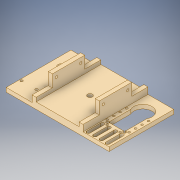
# Autodesk Inventor part: База
Saved by Autodesk Inventor 2019 (Build 230136000, 136)
## iProperties
Created: 2019-08-15
Part Number: База
Material: Пластик АБС
Document SubType Name: Modeling
Designer: Петров Иван
Density: 1.06 g/cm^3
Appearance: Гладкий — серовато-белый
Author: Петров Иван
Autodesk Inventor part; units mm, degrees
ref_plane "YZ Plane" through (0, 0, 0) normal (1, 0, 0) x (0, 1, 0)
ref_plane "XZ Plane" through (0, 0, 0) normal (0, 1, 0) x (-1, 0, 0)
ref_plane "XY Plane" through (0, 0, 0) normal (0, 0, 1) x (1, 0, 0)
sketch "Эскиз1" plane through (0, 0, 0) normal (0, 1, 0) x (-1, 0, 0)
  line L0 (-31.5, 40) -> (31.5, 40)
  line L1 (31.5, 40) -> (31.5, -40)
  line L2 (31.5, -40) -> (-31.5, -40)
  line L3 (-31.5, -40) -> (-31.5, 40)
  line L4 (-31.5, 40) -> (31.5, -40) construction
  line L5 (31.5, 40) -> (-31.5, -40) construction
  point P0 (0, 0)
  dimension "d0" = 63
  dimension "d1" = 80
  constraints: 12 end point, 2 midpoint, 2 parallel, 1 horizontal, 1 perpendicular
  measures "d0" distance of L1.end L2.end
  measures "d1" distance of L0.end L1.end
extrude "Выдавливание1" add sketch "Эскиз1" along normal blind 8
sketch "Эскиз2" plane through (0, 8, 0) normal (0, 1, 0) x (1, 0, 0)
  line L0 (-31.5, -40) -> (31.5, -40) projected
  line L1 (31.5, 40) -> (-31.5, 40) projected
  line L2 (-31.5, -40) -> (-26.5, -40)
  line L3 (-26.5, -40) -> (-26.5, 40)
  line L4 (-26.5, 40) -> (-31.5, 40)
  line L5 (-31.5, 40) -> (-31.5, -40)
  line L6 (31.5, -40) -> (31.5, 40) projected
  line L7 (31.5, 40) -> (26.5, 40)
  line L8 (26.5, 40) -> (26.5, -40)
  line L9 (26.5, -40) -> (31.5, -40)
  line L10 (31.5, -40) -> (31.5, 40)
  point P0 (0, 0)
  dimension "d4" = 5
  dimension "d5" = 5
  constraints: 16 end point, 4 parallel, 2 horizontal, 2 perpendicular, 2 point on line
  measures "d4" distance of L4.end L3.end
  measures "d5" distance of L9.end L8.end
extrude "Выдавливание2" add sketch "Эскиз2" along normal blind 20 contours L5 L1 L3 L0 | L8 L1 L6 L0
sketch "Эскиз3" plane through (-26.5, 8, 40) normal (1, 0, 0) x (0, 0, -1)
  line L0 (0, 0) -> (0, 20) projected
  line L1 (0, 0) -> (25, 0)
  line L2 (25, 0) -> (25, 14)
  line L3 (25, 14) -> (0, 14)
  line L4 (0, 14) -> (0, 0)
  circle A0 centre (25, 14) radius 1.5
  line L5 (80, 20) -> (0, 20) projected
  line L6 (40, 20) -> (40, 22.577)
  circle A1 centre (55, 14) radius 1.5
  point P0 (40, -8)
  dimension "d8" = 25
  dimension "d9" = 14
  dimension "d10" = 3
  constraints: 10 end point, 2 centre point, 2 parallel, 1 coincident, 1 horizontal, 1 midpoint, 1 perpendicular, 1 symmetric about line, 1 vertical, 1 other
  measures "d8" distance of L3.end L2.end
  measures "d9" distance of L2.end L1.end
  measures "d10" diameter of A0
extrude "Выдавливание3" cut sketch "Эскиз3" along normal blind 63.5 and the other way blind 5 contours A0 L2 L3 | L3 L2 A0 | A1
sketch "Эскиз4" plane through (0, 0, 0) normal (0, -1, 0) x (1, 0, 0)
  line L0 (31.5, -40) -> (31.5, 40) projected
  line L1 (31.5, -40) -> (63.5, -40)
  line L2 (63.5, -40) -> (63.5, 40)
  line L3 (63.5, 40) -> (31.5, 40)
  line L4 (31.5, 40) -> (31.5, -40)
  point P0 (0, 0)
  dimension "d15" = 32
  dimension "d16" = 80
  constraints: 8 end point, 2 parallel, 1 horizontal, 1 perpendicular
  measures "d15" distance of L3.end L2.end
  measures "d16" distance of L2.end L1.end
extrude "Выдавливание4" add sketch "Эскиз4" against normal blind 5
sketch "Эскиз5" plane through (0, 5, 0) normal (0, 1, 0) x (1, 0, 0)
  line L0 (34.2298, 0.6569) -> (31.9298, 0.6569)
  line L1 (34.2298, 0.6569) -> (34.2298, -0.7431)
  line L2 (31.9298, -0.7431) -> (34.2298, -0.7431)
  line L3 (31.9298, -7.3431) -> (31.9298, -0.7431)
  line L4 (34.2298, -7.3431) -> (31.9298, -7.3431)
  circle A0 centre (46.8802, 18.4564) radius 9.15
  circle A1 centre (46.8298, 18.4569) radius 1.5
  circle A2 centre (54.8298, -17.5431) radius 1.3
  circle A3 centre (60.3298, -4.0431) radius 1.3
  circle A4 centre (60.3298, -12.0431) radius 1.3
  circle A5 centre (60.3298, 3.9569) radius 1.3
  circle A6 centre (60.3298, 11.9569) radius 1.3
  circle A7 centre (38.8298, -17.5431) radius 1.3
  circle A8 centre (33.3298, -4.0431) radius 1.3
  circle A9 centre (33.3298, -12.0431) radius 1.3
  circle A10 centre (33.3298, 3.9569) radius 1.3
  circle A11 centre (33.3298, 11.9569) radius 1.3
  line L5 (46.7298, 29.4767) -> (46.7298, 28.9365)
  line L6 (39.8298, 29.4767) -> (46.7298, 29.4767)
  arc A12 (39.8298, 29.4767) -> (39.0798, 29.4255) centre (39.8298, 23.9569) ccw
  line L7 (39.0798, 26.9569) -> (39.0798, 29.4255)
  arc A13 (37.3298, 25.2069) -> (39.0798, 26.9569) centre (37.3298, 26.9569) ccw
  line L8 (36.8298, 25.2069) -> (37.3298, 25.2069)
  line L9 (36.8298, -12.3493) -> (36.8298, 25.2069)
  arc A14 (36.8298, -12.3493) -> (37.2219, -13.0376) centre (37.6298, -12.3493) ccw
  arc A15 (37.2219, -13.0376) -> (37.8353, -13.6509) centre (36.3298, -14.5431) ccw
  arc A16 (37.8353, -13.6509) -> (38.5235, -14.0431) centre (38.5235, -13.2431) ccw
  line L10 (55.136, -14.0431) -> (38.5235, -14.0431)
  arc A17 (55.136, -14.0431) -> (55.8243, -13.6509) centre (55.136, -13.2431) ccw
  arc A18 (56.4376, -13.0376) -> (55.8243, -13.6509) centre (57.3298, -14.5431) ccw
  arc A19 (55.8243, -13.6509) -> (56.4376, -13.0376) centre (57.3298, -14.5431) ccw
  line L11 (35.5069, 25.2069) -> (36.8298, 25.2069)
  arc A20 (35.5069, 25.2069) -> (35.3298, 23.9569) centre (39.8376, 23.9558) ccw
  line L12 (35.3298, 23.9569) -> (35.3298, 16.4569)
  line L13 (34.2298, 16.4569) -> (35.3298, 16.4569)
  line L14 (34.2298, 15.2569) -> (34.2298, 16.4569)
  line L15 (31.9298, 15.2569) -> (34.2298, 15.2569)
  line L16 (31.9298, 8.6569) -> (31.9298, 15.2569)
  line L17 (34.2298, 8.6569) -> (31.9298, 8.6569)
  line L18 (34.2298, 7.2569) -> (34.2298, 8.6569)
  line L19 (31.9298, 7.2569) -> (34.2298, 7.2569)
  line L20 (31.9298, 0.6569) -> (31.9298, 7.2569)
  line L21 (34.2298, 0.6569) -> (31.9298, 0.6569)
  line L22 (34.2298, -0.7431) -> (34.2298, 0.6569)
  line L23 (31.9298, -0.7431) -> (34.2298, -0.7431)
  line L24 (31.9298, -7.3431) -> (31.9298, -0.7431)
  line L25 (34.2298, -7.3431) -> (31.9298, -7.3431)
  line L26 (34.2298, -8.7431) -> (34.2298, -7.3431)
  line L27 (31.9298, -8.7431) -> (34.2298, -8.7431)
  line L28 (31.9298, -15.3431) -> (31.9298, -8.7431)
  line L29 (34.2298, -15.3431) -> (31.9298, -15.3431)
  line L30 (34.2298, -16.5629) -> (34.2298, -15.3431)
  arc A21 (34.2298, -16.5629) -> (34.31, -16.6431) centre (35.3298, -15.5431) ccw
  line L31 (35.5298, -16.6431) -> (34.31, -16.6431)
  line L32 (35.5298, -18.9431) -> (35.5298, -16.6431)
  line L33 (42.1298, -18.9431) -> (35.5298, -18.9431)
  line L34 (42.1298, -16.6431) -> (42.1298, -18.9431)
  line L35 (51.5298, -16.6431) -> (42.1298, -16.6431)
  line L36 (51.5298, -18.9431) -> (51.5298, -16.6431)
  line L37 (58.1298, -18.9431) -> (51.5298, -18.9431)
  line L38 (58.1298, -16.6431) -> (58.1298, -18.9431)
  line L39 (59.3496, -16.6431) -> (58.1298, -16.6431)
  arc A22 (59.3496, -16.6431) -> (59.4298, -16.5629) centre (58.3298, -15.5431) ccw
  line L40 (59.4298, -15.3431) -> (59.4298, -16.5629)
  line L41 (61.7298, -15.3431) -> (59.4298, -15.3431)
  line L42 (61.7298, -8.7431) -> (61.7298, -15.3431)
  line L43 (59.4298, -8.7431) -> (61.7298, -8.7431)
  line L44 (59.4298, -7.3431) -> (59.4298, -8.7431)
  line L45 (61.7298, -7.3431) -> (59.4298, -7.3431)
  line L46 (61.7298, -0.7431) -> (61.7298, -7.3431)
  line L47 (59.4298, -0.7431) -> (61.7298, -0.7431)
  line L48 (59.4298, 0.6569) -> (59.4298, -0.7431)
  line L49 (61.7298, 0.6569) -> (59.4298, 0.6569)
  line L50 (61.7298, 7.2569) -> (61.7298, 0.6569)
  line L51 (59.4298, 7.2569) -> (61.7298, 7.2569)
  line L52 (59.4298, 8.6569) -> (59.4298, 7.2569)
  line L53 (61.7298, 8.6569) -> (59.4298, 8.6569)
  line L54 (61.7298, 15.2568) -> (61.7298, 8.6569)
  line L55 (59.4305, 15.2569) -> (61.7298, 15.2568)
  line L56 (59.4306, 16.4569) -> (59.4305, 15.2569)
  line L57 (58.3306, 16.4569) -> (59.4306, 16.4569)
  line L58 (58.3308, 23.9569) -> (58.3306, 16.4569)
  arc A23 (58.3308, 23.9569) -> (58.1537, 25.2069) centre (53.8229, 23.9559) ccw
  line L59 (56.8308, 25.2069) -> (58.1537, 25.2069)
  line L60 (56.3308, 25.2069) -> (56.8308, 25.2069)
  arc A24 (54.5808, 26.957) -> (56.3308, 25.2069) centre (56.3308, 26.9569) ccw
  line L61 (54.5809, 29.4256) -> (54.5808, 26.957)
  arc A25 (54.5809, 29.4256) -> (53.8309, 29.4768) centre (53.8308, 23.957) ccw
  line L62 (46.9309, 29.477) -> (53.8309, 29.4768)
  line L63 (46.9309, 28.9368) -> (46.9309, 29.477)
  arc A26 (37.8353, -13.6509) -> (37.2219, -13.0376) centre (36.3298, -14.5431) ccw
  arc A27 (56.4376, -13.0376) -> (56.8298, -12.3493) centre (56.0298, -12.3493) ccw
  line L64 (56.8308, 25.2069) -> (56.8298, -12.3493)
  line L65 (56.0298, 18.3651) -> (56.8306, 18.3651)
  line L66 (37.7307, 18.3656) -> (36.8298, 18.3657)
  point P0 (0, 0)
  constraints: 134 end point, 34 point on circle, 28 centre point, 4 point on line, 1 perpendicular
extrude "Выдавливание5" cut sketch "Эскиз5" against normal through all contours L66 A0 L65 L64 A27 A18 A17 L10 A16 A26 A14 L9 | A0 | A26 A15 | A19 A18 | A1 | A2 | A3 | A4 | A5 | A6 | A7 | A8 | A9 | A10 | A11
sketch "Эскиз6" plane through (0, 5, 0) normal (0, 1, 0) x (1, 0, 0)
  arc A0 (56.0298, 18.3651) -> (37.7307, 18.3656) centre (46.8802, 18.4564) ccw projected
  circle A1 centre (46.8802, 18.4564) radius 11.25
  point P0 (0, 0)
  dimension "d21" = 22.5
  constraints: 1 centre point, 1 coincident
  measures "d21" diameter of A1
extrude "Выдавливание6" cut sketch "Эскиз6" against normal through all
sketch "Эскиз7" plane through (0, 8, 0) normal (0, 1, 0) x (1, 0, 0)
  circle A0 centre (0, 0) radius 3
  dimension "d24" = 6
  constraints: 1 centre point, 1 coincident
  measures "d24" diameter of A0
extrude "Выдавливание7" cut sketch "Эскиз7" against normal through all
sketch "Эскиз8" plane through (0, 5, 0) normal (0, 1, 0) x (1, 0, 0)
  line L0 (35.0061, -36.862) -> (35.0061, -19.4602) construction
  line L1 (37.1061, -36.862) -> (37.1061, -19.4602)
  line L2 (32.9061, -19.4602) -> (32.9061, -36.862)
  arc A0 (32.9061, -36.862) -> (37.1061, -36.862) centre (35.0061, -36.862) ccw
  arc A1 (37.1061, -19.4602) -> (32.9061, -19.4602) centre (35.0061, -19.4602) ccw
  line L3 (42.7556, -36.862) -> (42.7556, -19.46) construction
  line L4 (44.8556, -36.862) -> (44.8556, -19.46)
  line L5 (40.6556, -19.46) -> (40.6556, -36.862)
  arc A2 (40.6556, -36.862) -> (44.8556, -36.862) centre (42.7556, -36.862) ccw
  arc A3 (44.8556, -19.46) -> (40.6556, -19.46) centre (42.7556, -19.46) ccw
  line L6 (50.9531, -36.862) -> (50.9531, -19.46) construction
  line L7 (53.0949, -36.862) -> (53.0949, -19.46)
  line L8 (48.8113, -19.46) -> (48.8113, -36.862)
  arc A4 (48.8113, -36.862) -> (53.0949, -36.862) centre (50.9531, -36.862) ccw
  arc A5 (53.0949, -19.46) -> (48.8113, -19.46) centre (50.9531, -19.46) ccw
  line L9 (58.61, -36.862) -> (58.61, -19.46) construction
  line L10 (60.7604, -36.862) -> (60.7604, -19.46)
  line L11 (56.4597, -19.46) -> (56.4597, -36.862)
  arc A6 (56.4597, -36.862) -> (60.7604, -36.862) centre (58.61, -36.862) ccw
  arc A7 (60.7604, -19.46) -> (56.4597, -19.46) centre (58.61, -19.46) ccw
  point P0 (0, 0)
  point P1 (35.0061, -28.1611)
  point P2 (42.7556, -28.161)
  point P3 (35.0061, -38.962)
  point P4 (42.7556, -38.962)
  point P5 (50.9531, -28.161)
  point P6 (58.61, -28.161)
  dimension "d27" = 4.2
  dimension "d28" = 4.2
  dimension "d29" = 17.402
  constraints: 32 end point, 18 point on circle, 16 tangent, 8 centre point, 6 parallel, 4 midpoint, 2 vertical, 1 horizontal alignment
  measures "d27" diameter of A1
  measures "d28" diameter of A3
  measures "d29" distance of L4.start L4.end
extrude "Выдавливание8" cut sketch "Эскиз8" against normal blind 19.25
sketch "Эскиз9" plane through (31.5, 28, 40) normal (1, 0, 0) x (0, 0, -1)
  line L0 (0, 0) -> (20, 0)
  line L1 (20, 0) -> (20, -15)
  line L2 (20, -15) -> (0, -15)
  line L3 (0, -15) -> (0, 0)
  line L4 (80, 0) -> (60, 0)
  line L5 (60, 0) -> (60, -15)
  line L6 (60, -15) -> (80, -15)
  line L7 (80, -15) -> (80, 0)
  point P0 (40, -28)
  dimension "d32" = 20
  dimension "d33" = 15
  dimension "d34" = 20
  dimension "d35" = 15
  constraints: 16 end point, 4 parallel, 2 horizontal, 2 perpendicular, 1 point on line
  measures "d32" distance of L1.end L2.end
  measures "d33" distance of L0.end L1.end
  measures "d34" distance of L6.end L5.end
  measures "d35" distance of L5.end L4.end
extrude "Выдавливание9" cut sketch "Эскиз9" against normal blind 71.25
sketch "Эскиз10" plane through (-31.5, 0, -40) normal (-1, 0, 0) x (0, 0, 1)
  line L0 (0, 0) -> (0, 13) projected
  line L1 (80, 5) -> (0, 5) projected
  line L2 (0, 0) -> (80, 0)
  line L3 (80, 0) -> (80, 5)
  line L4 (80, 5) -> (0, 5)
  line L5 (0, 5) -> (0, 0)
  point P0 (40, 0)
  constraints: 8 end point, 2 parallel, 1 horizontal, 1 perpendicular
extrude "Выдавливание10" add sketch "Эскиз10" along normal blind 32
sketch "Эскиз12" plane through (-31.5, 5, 40) normal (0, 1, 0) x (1, 0, 0)
  circle A0 centre (-20.5991, 65.4688) radius 1.5
  circle A1 centre (-11.0978, 16.5688) radius 1.5
  circle A2 centre (-29.5417, 16.5688) radius 1.5
  line L0 (-32.0417, 43.6688) -> (-32.0417, 14.0688)
  line L1 (-8.5978, 14.0688) -> (-32.0417, 14.0688)
  line L2 (-8.5978, 14.0688) -> (-8.5978, 51.7665)
  line L3 (-8.5978, 51.7665) -> (-5.622, 51.7665)
  line L4 (-5.622, 51.7665) -> (-5.622, 61.4688)
  line L5 (-5.622, 61.4688) -> (-16.5991, 61.4688)
  line L6 (-16.5991, 61.4688) -> (-16.5991, 69.4688)
  line L7 (-16.5991, 69.4688) -> (-24.5991, 69.4688)
  line L8 (-24.5991, 69.4688) -> (-24.5991, 61.4688)
  line L9 (-24.5991, 61.4688) -> (-35.422, 61.4688)
  line L10 (-35.422, 61.4688) -> (-40.422, 61.4688)
  line L11 (-40.422, 61.4688) -> (-40.422, 48.6688)
  line L12 (-35.422, 43.6688) -> (-40.422, 48.6688)
  line L13 (-35.422, 43.6688) -> (-32.0417, 43.6688)
  circle A3 centre (-20.522, 56.4688) radius 4
  line L14 (-10.4717, 49.3901) -> (-10.522, 49.2688)
  line L15 (-10.522, 49.2688) -> (-10.522, 25.6626)
  arc A4 (-10.9141, 24.9743) -> (-10.522, 25.6626) centre (-11.322, 25.6626) ccw
  arc A5 (-10.9141, 24.9743) -> (-11.5275, 24.361) centre (-10.022, 23.4688) ccw
  arc A6 (-12.2157, 23.9688) -> (-11.5275, 24.361) centre (-12.2157, 24.7688) ccw
  line L16 (-12.2157, 23.9688) -> (-28.8282, 23.9688)
  arc A7 (-29.5165, 24.361) -> (-28.8282, 23.9688) centre (-28.8282, 24.7688) ccw
  arc A8 (-29.5165, 24.361) -> (-30.1298, 24.9743) centre (-31.022, 23.4688) ccw
  arc A9 (-30.522, 25.6626) -> (-30.1298, 24.9743) centre (-29.722, 25.6626) ccw
  line L17 (-30.522, 25.6626) -> (-30.522, 44.6671)
  arc A10 (-30.522, 44.6671) -> (-30.5274, 44.9956) centre (-40.522, 44.6671) ccw
  line L18 (-26.1915, 51.4688) -> (-30.5274, 44.9956)
  line L19 (-26.1915, 51.4688) -> (-11.8607, 51.4688)
  line L20 (-10.4717, 49.3901) -> (-11.8607, 51.4688)
  circle A11 centre (-34.022, 49.9688) radius 1.3
  circle A12 centre (-28.522, 20.4688) radius 1.3
  circle A13 centre (-12.522, 20.4688) radius 1.3
  line L21 (-7.922, 45.2688) -> (-5.622, 45.2688)
  line L22 (-7.922, 46.6688) -> (-7.922, 45.2688)
  line L23 (-5.622, 46.6688) -> (-7.922, 46.6688)
  line L24 (-5.622, 51.7665) -> (-5.622, 46.6688)
  line L25 (-8.5978, 51.7665) -> (-5.622, 51.7665)
  line L26 (-8.5978, 19.0688) -> (-8.5978, 51.7665)
  line L27 (-5.622, 19.0688) -> (-8.5978, 19.0688)
  line L28 (-5.622, 45.2688) -> (-5.622, 19.0688)
  circle A14 centre (-7.022, 41.9688) radius 1.3
  circle A15 centre (-7.022, 25.9688) radius 1.3
  circle A16 centre (-7.022, 33.9688) radius 1.3
  circle A17 centre (-7.022, 49.9688) radius 1.3
  circle A18 centre (-34.022, 41.9688) radius 1.3
  circle A19 centre (-34.022, 25.9688) radius 1.3
  circle A20 centre (-34.022, 33.9688) radius 1.3
  line L29 (-32.0417, 19.0688) -> (-35.422, 19.0688)
  line L30 (-32.0417, 43.6688) -> (-32.0417, 19.0688)
  line L31 (-35.422, 43.6688) -> (-32.0417, 43.6688)
  line L32 (-35.422, 19.0688) -> (-35.422, 43.6688)
  line L33 (-35.422, 61.4688) -> (-35.422, 66.4688)
  line L34 (-35.422, 66.4688) -> (-40.422, 66.4688)
  line L35 (-40.422, 66.4688) -> (-40.422, 61.4688)
  line L36 (-35.422, 61.4688) -> (-40.422, 61.4688)
  line L37 (-35.422, 66.4688) -> (-40.422, 66.4688)
  line L38 (-35.422, 66.4688) -> (-40.422, 66.4688)
  line L39 (-35.422, 66.4688) -> (-35.422, 68.6688)
  line L40 (-35.422, 68.6688) -> (-40.422, 68.6688)
  line L41 (-40.422, 68.6688) -> (-40.422, 66.4688)
  point P0 (31.5, 40)
  constraints: 84 end point, 21 centre point, 14 point on circle
extrude "Выдавливание12" cut sketch "Эскиз12" against normal blind 10 contours A0 | A1 | A2 | A3
